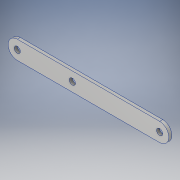
# Autodesk Inventor part: CLB_079_ClimberMountReinforceBar
Saved by Autodesk Inventor 2018.3 (Build 223284000, 284)
## iProperties
Created: 2020-03-04
Part Number: CLB_079_ClimberMountReinforceBar
Material: Aluminum 6061
Document SubType Name: Modeling
Designer: myerpaul
Density: 2.7 g/cm^3
Appearance: Aluminum - Flat
Author: myerpaul
Autodesk Inventor part; units mm, degrees
ref_plane "YZ Plane" through (0, 0, 0) normal (1, 0, 0) x (0, 1, 0)
ref_plane "XZ Plane" through (0, 0, 0) normal (0, 1, 0) x (-1, 0, 0)
ref_plane "XY Plane" through (0, 0, 0) normal (0, 0, 1) x (1, 0, 0)
sketch "Sketch1" plane through (0, 0, 0) normal (0, 0, 1) x (1, 0, 0)
  line L0 (0, 0) -> (147.701, 0) construction
  line L1 (0, -9.525) -> (147.701, -9.525)
  line L2 (147.701, 9.525) -> (0, 9.525)
  arc A0 (0, 9.525) -> (0, -9.525) centre (0, 0) ccw
  arc A1 (147.701, -9.525) -> (147.701, 9.525) centre (147.701, 0) ccw
  point P0 (57.15, 0)
  dimension "d0" = 19.05
  dimension "d5" = 57.15
  dimension "d6" = 90.551
  constraints: 8 end point, 4 point on circle, 4 tangent, 2 centre point, 2 coincident, 1 horizontal, 1 parallel, 1 point on line
  measures "d0" diameter of A0
  measures "d5" distance of point (57.15, 0) point (0, 0)
  measures "d6" distance of L0.end point (57.15, 0)
extrude "Extrusion1" add sketch "Sketch1" along normal blind 3.175
hole "Hole1" at (0, 0, 0) at (147.701, 0, 0) at (57.15, 0, 0) direction (0, 0, 1) diameter 6.35 end through all
body "Solid1"
